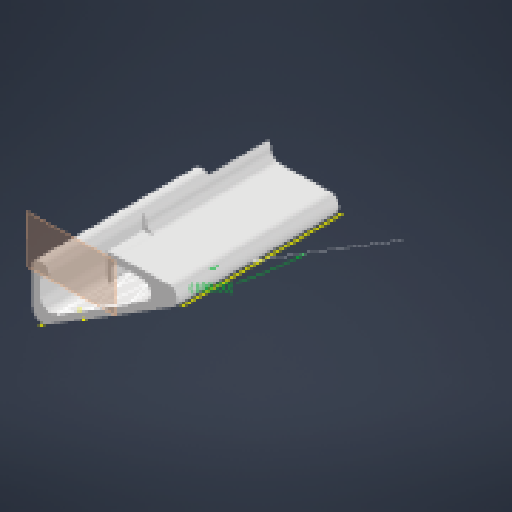
# Autodesk Inventor part: PiHoldertoScreenMount
Saved by Autodesk Inventor 2023 (Build 270158000, 158)
## iProperties
Created: 2023-02-23
Part Number: PiHoldertoScreenMount
Material: Generic
Document SubType Name: Modeling
Designer: uzair
Density: 1 g/cm^3
Appearance: Default
Author: uzair
Autodesk Inventor part; units mm, degrees
ref_plane "YZ Plane" through (0, 0, 0) normal (1, 0, 0) x (0, 1, 0)
ref_plane "XZ Plane" through (0, 0, 0) normal (0, 1, 0) x (-1, 0, 0)
ref_plane "XY Plane" through (0, 0, 0) normal (0, 0, 1) x (1, 0, 0)
ref_plane "Work Plane1" through (8.0832, -1.7479, 0.0018) normal (0.0000225, 0.0000002, 1) x (0.9997665, 0.0216087, -0.0000225)
sketch "Sketch1" plane through (8.0832, -1.7479, 0.0018) normal (0.0000225, 0.0000002, 1) x (0.9997665, 0.0216087, -0.0000225)
  line L0 (21.1769, -11.5228) -> (-21.1769, -11.5228)
  line L1 (-21.1769, -11.5228) -> (-21.1769, 11.5228)
  line L2 (-21.1769, 11.5228) -> (21.1769, 11.5228)
  line L3 (21.1769, 11.5228) -> (21.1769, -11.5228)
  line L4 (-21.1769, -11.5228) -> (-21.1769, -36.5228)
  line L5 (-21.1769, -11.5228) -> (3.8231, -11.5228) construction
  line L6 (-21.1769, -36.5228) -> (21.1769, -11.5228)
  line L7 (64.5473, 11.7548) -> (-20.1602, -38.2452)
  line L8 (-20.1602, -38.2452) -> (-22.1935, -34.8005)
  line L9 (-22.1935, -34.8005) -> (62.514, 15.1995)
  line L10 (62.514, 15.1995) -> (64.5473, 11.7548)
  line L11 (64.5473, 11.7548) -> (-22.1935, -34.8005) construction
  line L12 (-20.1602, -38.2452) -> (62.514, 15.1995) construction
  line L13 (62.514, 15.1995) -> (21.1769, 15.1995)
  line L14 (21.1769, 15.1995) -> (21.1769, 11.1995)
  line L15 (21.1769, 11.1995) -> (62.514, 11.1995)
  line L16 (62.514, 11.1995) -> (62.514, 15.1995)
  line L17 (-21.1769, -36.5228) -> (-17.1769, -36.5228)
  line L18 (-17.1769, -36.5228) -> (-17.1769, -11.5228)
  line L19 (-17.1769, -11.5228) -> (-21.1769, -11.5228)
  line L20 (-21.1769, -11.5228) -> (-21.1769, -36.5228)
  line L21 (62.514, 15.1995) -> (21.1769, -9.2004)
  line L22 (17.2423, -11.5228) -> (-17.1769, -31.8393)
  line L23 (-17.1769, -11.5228) -> (17.2423, -11.5228)
  line L24 (21.1769, -9.2004) -> (21.1769, 11.1995)
  line L25 (55.7374, 11.1995) -> (21.1769, 11.1995)
  line L26 (21.1769, 14.8544) -> (62.514, 15.1995)
  point P0 (-8.0436, 1.9222)
  point P1 (-17.1769, -31.8393)
  point P2 (-17.1769, -11.5228)
  dimension "d1" = 25
  dimension "d2" = 90
  dimension "d3" = 4
  dimension "d4" = 4
  dimension "d5" = 4
  constraints: 54 end point, 11 point on line, 9 parallel, 6 perpendicular, 4 horizontal, 2 collinear, 2 midpoint, 1 vertical
  measures "d1" distance of L0.end L4.end
  measures "d2" angle of L4 L5
  measures "d3" distance of L7.end L8.end
  measures "d4" distance of L14.end L13.end
  measures "d5" distance of L19.end L18.end
extrude "Extrusion1" add sketch "Sketch1" against normal blind 86.14 contours L6 L18 L9 L0 | L0 L9 L3 | L3 L9 L15 L16 L10 L7 L18 L6 | L18 L7 L17 L6 | L6 L4 L9 L18 | L18 L9 L4 L0 | L3 L14 L26 L9 L15 | L9 L16 L15 | L17 L7 L8 | L26 L14 L13
fillet "Fillet1" radius 5 6 edges at (70.2532, 14.7989, -43.0696) (72.3604, 11.399, -43.0696) (63.5646, 10.6534, -43.0694) (-8.4026, -33.951, -43.0678) (-11.2469, -40.4198, -43.0677) (-12.3005, -38.7198, -43.0677)
sketch "Sketch2" plane through (-4.8076, -36.4282, -86.1379) normal (0.526809, -0.8499837, -0.0000117) x (0.8499837, 0.526809, -0.0000193)
  line L0 (84.2561, 86.14) -> (84.2561, 0) projected
  line L1 (84.2561, 43.07) -> (-5, 43.07)
  line L2 (-5, 86.14) -> (-5, 0) projected
  line L3 (84.2561, 43.07) -> (173.5122, 43.07) construction
  point P0 (23.2755, 86.138)
  dimension "d9" = 180
  constraints: 4 end point, 2 midpoint, 1 collinear, 1 horizontal
  measures "d9" angle of L1 L3
sketch "Sketch3" plane through (-0.958, -29.3375, 0.002) normal (-0.526809, 0.8499837, 0.0000117) x (0.8499837, 0.526809, -0.0000193)
  line L0 (46.1491, 0) -> (46.1491, 86.14) projected
  line L1 (1.5699, 0) -> (1.5699, 86.14) projected
  line L2 (46.1491, 86.14) -> (1.5699, 86.14)
  line L3 (1.5699, 86.14) -> (1.5699, 0)
  line L4 (1.5699, 0) -> (46.1491, 0)
  line L5 (46.1491, 0) -> (46.1491, 86.14)
  line L6 (0, 86.14) -> (57.6045, 86.14) projected
  line L7 (23.8595, 86.14) -> (46.1491, 43.07)
  line L8 (46.1491, 86.14) -> (48.1824, 86.14) projected
  line L9 (46.1491, 86.14) -> (1.5699, 0)
  line L10 (-1.8748, 86.14) -> (1.5699, 86.14) projected
  line L11 (46.1491, 0) -> (1.5699, 86.14)
  line L12 (23.8595, 86.14) -> (1.5699, 43.07)
  line L13 (23.8595, 0) -> (1.5699, 43.07)
  line L14 (46.1491, 43.07) -> (23.8595, 0)
  point P0 (16.2696, 0.002)
  point P1 (35.0043, 64.605)
  point P2 (35.0043, 21.535)
  point P3 (12.7147, 21.535)
  point P4 (12.7147, 64.605)
  constraints: 20 end point, 7 midpoint, 4 parallel, 2 point on line, 1 horizontal, 1 perpendicular
sketch "Sketch4" plane through (-0.958, -29.3375, 0.002) normal (-0.526809, 0.8499837, 0.0000117) x (0.8499837, 0.526809, -0.0000193)
  point P0 (35.0043, 64.605)
  point P1 (35.0043, 21.535)
  point P2 (12.7147, 21.535)
  point P3 (12.7147, 64.605)
hole "Hole1" at (28.7936, -10.8969, -64.6036) at (28.7946, -10.8969, -21.5336) at (9.8488, -22.6393, -21.5332) at (9.8478, -22.6393, -64.6032) direction (0.526809, -0.8499837, -0.0000117) diameter 3.4 end through all
sketch "Sketch7" plane through (8.0832, -1.7479, 0.0018) normal (0.0000225, 0.0000002, 1) x (0.9997665, 0.0216087, -0.0000225)
  line L0 (37.4303, 11.1995) -> (21.1769, 11.1995) projected
  line L1 (21.1769, 11.1995) -> (19.5026, 11.1995)
  line L2 (19.5026, 11.1995) -> (19.5026, 23.073)
  line L3 (19.5026, 23.073) -> (21.1769, 23.073)
  line L4 (21.1769, 23.073) -> (21.1769, 11.1995)
  line L5 (-11.8904, -11.8459) -> (-21.1768, -11.8459)
  line L6 (-21.1768, -11.8459) -> (-21.1768, -6.8459)
  line L7 (-21.1768, -6.8459) -> (-11.8904, -6.8459)
  line L8 (-11.8904, -6.8459) -> (-11.8904, -11.8459)
  line L9 (21.1769, 11.1995) -> (21.1769, 15.1995) projected
  line L10 (21.1769, 11.1995) -> (19.5026, 11.1995)
  line L11 (19.5026, 11.1995) -> (19.5026, 0.0092)
  line L12 (19.5026, 0.0092) -> (21.1769, 0.0092)
  line L13 (21.1769, 0.0092) -> (21.1769, 11.1995)
  point P0 (-8.0436, 1.9222)
  point P1 (19.5026, 11.1995)
  dimension "d26" = 5
  constraints: 24 end point, 6 parallel, 3 horizontal, 3 perpendicular
  measures "d26" distance of L5.end L6.end
extrude "Extrusion4" add sketch "Sketch7" against normal blind 86.14
fillet "Fillet3" radius 4 7 edges at (28.9257, 13.9057, -43.0687) (28.7556, 21.7773, -43.0687) (-8.8347, -13.9622, -43.0678) (-3.6574, -8.8491, -43.0679) (-12.9417, -9.0498, -43.0677) (29.0122, 9.9066, -43.0687) (29.254, -1.2811, -43.0687)
sketch "Sketch9" plane through (8.0832, -1.7479, 0.0018) normal (0.0000225, 0.0000002, 1) x (0.9997665, 0.0216087, -0.0000225)
  line L0 (19.5026, 0.0092) -> (19.5026, 23.073) projected
  line L1 (19.5026, 14.8472) -> (24.5026, 14.8472)
  line L2 (25.1769, 15.1995) -> (52.076, 15.1995) projected
  line L3 (19.5026, 14.8472) -> (24.5026, 14.8472) construction
  line L4 (19.5026, 23.073) -> (24.5026, 23.073)
  line L5 (24.5026, 23.073) -> (24.5026, 14.8472)
  line L6 (24.5026, 14.8472) -> (19.5026, 14.8472)
  line L7 (19.5026, 14.8472) -> (19.5026, 23.073)
  point P0 (-8.0436, 1.9222)
  dimension "d33" = 5
  dimension "d34" = 0
  constraints: 12 end point, 3 parallel, 2 horizontal, 1 collinear, 1 perpendicular, 1 point on line
  measures "d33" distance of L1.start L1.end
  measures "d34" distance between parallel lines of L1 L3
extrude "Extrusion6" cut sketch "Sketch9" against normal blind 19.224
fillet "Fillet6" radius 5 2 edges at (32.2502, 14.0347, -9.6107) (32.2591, 13.6253, -9.6107)
body "Solid1"
